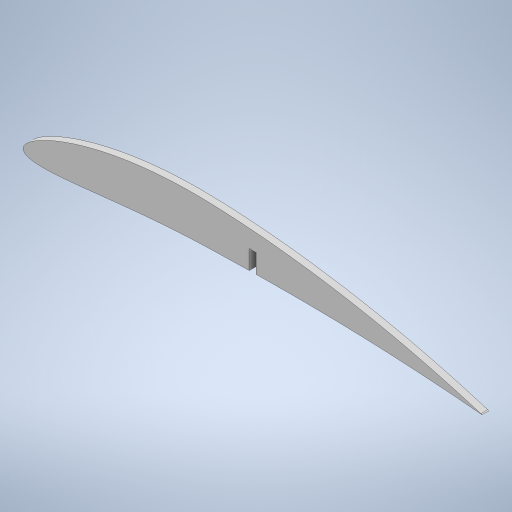
# Autodesk Inventor part: 6409_v1
Saved by Autodesk Inventor 2023 (Build 270158000, 158)
## iProperties
Created: 2023-03-24
Part Number: 6409_v1
Material: 一般
Document SubType Name: Modeling
Designer: USER
Density: 1 g/cm^3
Appearance: 預設
Author: USER
Autodesk Inventor part; units mm, degrees
ref_plane "YZ Plane" through (0, 0, 0) normal (1, 0, 0) x (0, 1, 0)
ref_plane "XZ Plane" through (0, 0, 0) normal (0, 1, 0) x (-1, 0, 0)
ref_plane "XY Plane" through (0, 0, 0) normal (0, 0, 1) x (1, 0, 0)
sketch "草圖1" plane through (0, 0, 0) normal (0, 0, 1) x (1, 0, 0)
  line L0 (0, 0) -> (200, 0)
  line L1 (199.444, 0.05) -> (200, 0)
  line L2 (199.464, 0.168) -> (200, 0)
  spline S0 degree 5 poles (199.464, 0.168) (199.4095, 0.1835) (199.2336, 0.2336) (198.9218, 0.3242) (198.496, 0.4567) (197.962, 0.6342) (197.287, 0.8521) (196.4984, 1.0928) (195.6233, 1.3514) (194.7061, 1.6209) (193.7762, 1.8964) (192.8362, 2.177) (191.8768, 2.4631) (190.8844, 2.7561) (189.8526, 3.0561) (188.7833, 3.3625) (187.6822, 3.6741) (186.5571, 3.9893) (185.4138, 4.3073) (184.2543, 4.6272) (183.0784, 4.9491) (181.8846, 5.2728) (180.6711, 5.5984) (179.4371, 5.9257) (178.183, 6.2543) (176.9101, 6.5838) (175.6203, 6.9137) (174.3152, 7.2433) (172.9962, 7.5724) (171.664, 7.9007) (170.319, 8.2281) (168.9611, 8.5544) (167.5902, 8.8796) (166.2063, 9.2036) (164.8097, 9.5262) (163.4007, 9.8473) (161.9799, 10.1664) (160.548, 10.4834) (159.1056, 10.798) (157.6531, 11.11) (156.1909, 11.4191) (154.7194, 11.7252) (153.2387, 12.0283) (151.7491, 12.3283) (150.2507, 12.6249) (148.7438, 12.9182) (147.2286, 13.208) (145.7054, 13.4942) (144.1748, 13.7765) (142.6369, 14.0549) (141.0922, 14.3291) (139.541, 14.5991) (137.9837, 14.8646) (136.4204, 15.1257) (134.8513, 15.3821) (133.2768, 15.6338) (131.6969, 15.8807) (130.1119, 16.1228) (128.5219, 16.3598) (126.9272, 16.5917) (125.328, 16.8185) (123.7244, 17.04) (122.1167, 17.256) (120.5053, 17.4666) (118.8902, 17.6716) (117.272, 17.871) (115.6509, 18.0647) (114.0273, 18.2527) (112.4014, 18.4349) (110.7734, 18.6112) (109.1437, 18.7814) (107.5123, 18.9454) (105.8794, 19.103) (104.245, 19.2542) (102.6092, 19.3986) (100.9723, 19.5363) (99.3345, 19.6671) (97.6961, 19.7913) (96.0577, 19.9087) (94.4196, 20.0198) (92.7824, 20.1244) (91.1465, 20.2228) (89.5119, 20.3148) (87.8788, 20.4002) (86.2468, 20.4787) (84.6155, 20.5496) (82.9845, 20.6124) (81.3534, 20.6662) (79.7218, 20.7103) (78.0897, 20.744) (76.4575, 20.7666) (74.8259, 20.7775) (73.1957, 20.7763) (71.5681, 20.7625) (69.9439, 20.7358) (68.3242, 20.696) (66.7097, 20.643) (65.1008, 20.5768) (63.4979, 20.4976) (61.9011, 20.4053) (60.3105, 20.3004) (58.7262, 20.1828) (57.1483, 20.0528) (55.5771, 19.9104) (54.0129, 19.7558) (52.4562, 19.5889) (50.9074, 19.4098) (49.3671, 19.2184) (47.8357, 19.0148) (46.3136, 18.7991) (44.8014, 18.5712) (43.2993, 18.3313) (41.8078, 18.0795) (40.3272, 17.816) (38.858, 17.5408) (37.4006, 17.2541) (35.9555, 16.9562) (34.5231, 16.6473) (33.1039, 16.3274) (31.6986, 15.9968) (30.3076, 15.6556) (28.9316, 15.304) (27.5711, 14.9419) (26.2267, 14.5696) (24.899, 14.1872) (23.5886, 13.7948) (22.2961, 13.3927) (21.0222, 12.9812) (19.7674, 12.5607) (18.5326, 12.1315) (17.3186, 11.6937) (16.1265, 11.2477) (14.9573, 10.7932) (13.8123, 10.3304) (12.6929, 9.8591) (11.6003, 9.3796) (10.5358, 8.8922) (9.5005, 8.3976) (8.4956, 7.8963) (7.5226, 7.3887) (6.5837, 6.8747) (5.6816, 6.3534) (4.8196, 5.8236) (4.0017, 5.2845) (3.2322, 4.7361) (2.5159, 4.1804) (1.8583, 3.6194) (1.2677, 3.0533) (0.7555, 2.4773) (0.3382, 1.8826) (0.0385, 1.2662) (-0.1096, 0.6422) (-0.0677, 0.0433) (0.1824, -0.4963) (0.6145, -0.9555) (1.1788, -1.3267) (1.8344, -1.6157) (2.5605, -1.8373) (3.3461, -2.0093) (4.1841, -2.1444) (5.0679, -2.2486) (5.9921, -2.3244) (6.9524, -2.3733) (7.9452, -2.3979) (8.968, -2.4011) (10.0186, -2.3861) (11.0953, -2.3557) (12.1964, -2.3118) (13.3204, -2.2555) (14.4661, -2.1876) (15.6322, -2.1089) (16.8177, -2.0202) (18.0217, -1.9223) (19.2436, -1.8164) (20.4826, -1.7033) (21.738, -1.584) (23.0091, -1.4593) (24.2952, -1.3298) (25.5956, -1.1961) (26.9095, -1.0586) (28.2365, -0.9178) (29.5761, -0.7742) (30.9277, -0.6281) (32.2912, -0.48) (33.6662, -0.3303) (35.0524, -0.1793) (36.4495, -0.0276) (37.857, 0.1246) (39.2746, 0.2768) (40.7019, 0.4287) (42.1384, 0.5799) (43.5837, 0.73) (45.0375, 0.8788) (46.4996, 1.0258) (47.9697, 1.1707) (49.4477, 1.3133) (50.9332, 1.4531) (52.4262, 1.59) (53.9265, 1.7237) (55.4338, 1.854) (56.948, 1.9808) (58.4688, 2.1039) (59.9958, 2.223) (61.5288, 2.338) (63.0673, 2.4485) (64.6108, 2.5544) (66.1589, 2.6552) (67.7112, 2.7507) (69.2676, 2.8408) (70.8281, 2.9251) (72.3929, 3.0037) (73.9625, 3.0764) (75.5374, 3.1435) (77.1181, 3.2051) (78.7049, 3.2615) (80.2978, 3.3131) (81.8967, 3.3604) (83.5008, 3.4042) (85.1094, 3.445) (86.7214, 3.4836) (88.3359, 3.5204) (89.952, 3.556) (91.5692, 3.5905) (93.187, 3.6238) (94.8053, 3.6559) (96.424, 3.6864) (98.0432, 3.7151) (99.6629, 3.7415) (101.2831, 3.7654) (102.9037, 3.7868) (104.5245, 3.8056) (106.1452, 3.8217) (107.7654, 3.8353) (109.385, 3.8465) (111.0035, 3.8553) (112.6206, 3.8618) (114.2361, 3.8659) (115.8498, 3.8676) (117.4615, 3.8668) (119.0711, 3.8633) (120.6783, 3.8571) (122.2829, 3.8482) (123.8848, 3.8366) (125.4837, 3.8221) (127.0794, 3.805) (128.6716, 3.7851) (130.26, 3.7626) (131.8445, 3.7374) (133.4248, 3.7096) (135.0006, 3.6791) (136.5718, 3.646) (138.1379, 3.6102) (139.6989, 3.5718) (141.2543, 3.5307) (142.8039, 3.487) (144.3475, 3.4408) (145.8845, 3.3921) (147.4148, 3.3409) (148.9381, 3.2874) (150.454, 3.2316) (151.9623, 3.1735) (153.4627, 3.1132) (154.9551, 3.0506) (156.4392, 2.9857) (157.9145, 2.9187) (159.3809, 2.8495) (160.8377, 2.7784) (162.2844, 2.7053) (163.7204, 2.6305) (165.1452, 2.5541) (166.5583, 2.4763) (167.9594, 2.3969) (169.3483, 2.3162) (170.7249, 2.2339) (172.0891, 2.1502) (173.4403, 2.0649) (174.778, 1.9784) (176.1009, 1.8908) (177.4074, 1.8025) (178.6961, 1.714) (179.9659, 1.6254) (181.2162, 1.5369) (182.4477, 1.4482) (183.6617, 1.359) (184.8595, 1.2688) (186.0408, 1.1775) (187.2035, 1.0856) (188.3417, 0.9942) (189.4483, 0.9051) (190.5176, 0.8193) (191.5476, 0.7372) (192.5445, 0.6572) (193.521, 0.5757) (194.4856, 0.4907) (195.4358, 0.4023) (196.3428, 0.3174) (197.1637, 0.246) (197.8722, 0.1935) (198.4359, 0.1544) (198.8815, 0.1138) (199.2051, 0.0778) (199.3872, 0.0567) (199.444, 0.05) knots 0.005109 0.005109 0.005109 0.005109 0.005109 0.005109 0.006667 0.01 0.013333 0.016667 0.02 0.023333 0.026667 0.03 0.033333 0.036667 0.04 0.043333 0.046667 0.05 0.053333 0.056667 0.06 0.063333 0.066667 0.07 0.073333 0.076667 0.08 0.083333 0.086667 0.09 0.093333 0.096667 0.1 0.103333 0.106667 0.11 0.113333 0.116667 0.12 0.123333 0.126667 0.13 0.133333 0.136667 0.14 0.143333 0.146667 0.15 0.153333 0.156667 0.16 0.163333 0.166667 0.17 0.173333 0.176667 0.18 0.183333 0.186667 0.19 0.193333 0.196667 0.2 0.203333 0.206667 0.21 0.213333 0.216667 0.22 0.223333 0.226667 0.23 0.233333 0.236667 0.24 0.243333 0.246667 0.25 0.253333 0.256667 0.26 0.263333 0.266667 0.27 0.273333 0.276667 0.28 0.283333 0.286667 0.29 0.293333 0.296667 0.3 0.303333 0.306667 0.31 0.313333 0.316667 0.32 0.323333 0.326667 0.33 0.333333 0.336667 0.34 0.343333 0.346667 0.35 0.353333 0.356667 0.36 0.363333 0.366667 0.37 0.373333 0.376667 0.38 0.383333 0.386667 0.39 0.393333 0.396667 0.4 0.403333 0.406667 0.41 0.413333 0.416667 0.42 0.423333 0.426667 0.43 0.433333 0.436667 0.44 0.443333 0.446667 0.45 0.453333 0.456667 0.46 0.463333 0.466667 0.47 0.473333 0.476667 0.48 0.483333 0.486667 0.49 0.493333 0.496667 0.5 0.503333 0.506667 0.51 0.513333 0.516667 0.52 0.523333 0.526667 0.53 0.533333 0.536667 0.54 0.543333 0.546667 0.55 0.553333 0.556667 0.56 0.563333 0.566667 0.57 0.573333 0.576667 0.58 0.583333 0.586667 0.59 0.593333 0.596667 0.6 0.603333 0.606667 0.61 0.613333 0.616667 0.62 0.623333 0.626667 0.63 0.633333 0.636667 0.64 0.643333 0.646667 0.65 0.653333 0.656667 0.66 0.663333 0.666667 0.67 0.673333 0.676667 0.68 0.683333 0.686667 0.69 0.693333 0.696667 0.7 0.703333 0.706667 0.71 0.713333 0.716667 0.72 0.723333 0.726667 0.73 0.733333 0.736667 0.74 0.743333 0.746667 0.75 0.753333 0.756667 0.76 0.763333 0.766667 0.77 0.773333 0.776667 0.78 0.783333 0.786667 0.79 0.793333 0.796667 0.8 0.803333 0.806667 0.81 0.813333 0.816667 0.82 0.823333 0.826667 0.83 0.833333 0.836667 0.84 0.843333 0.846667 0.85 0.853333 0.856667 0.86 0.863333 0.866667 0.87 0.873333 0.876667 0.88 0.883333 0.886667 0.89 0.893333 0.896667 0.9 0.903333 0.906667 0.91 0.913333 0.916667 0.92 0.923333 0.926667 0.93 0.933333 0.936667 0.94 0.943333 0.946667 0.95 0.953333 0.956667 0.96 0.963333 0.966667 0.97 0.973333 0.976667 0.98 0.983333 0.986667 0.99 0.993333 0.994906 0.994906 0.994906 0.994906 0.994906 0.994906 weights 1 1 1 1 1 1 1 1 1 1 1 1 1 1 1 1 1 1 1 1 1 1 1 1 1 1 1 1 1 1 1 1 1 1 1 1 1 1 1 1 1 1 1 1 1 1 1 1 1 1 1 1 1 1 1 1 1 1 1 1 1 1 1 1 1 1 1 1 1 1 1 1 1 1 1 1 1 1 1 1 1 1 1 1 1 1 1 1 1 1 1 1 1 1 1 1 1 1 1 1 1 1 1 1 1 1 1 1 1 1 1 1 1 1 1 1 1 1 1 1 1 1 1 1 1 1 1 1 1 1 1 1 1 1 1 1 1 1 1 1 1 1 1 1 1 1 1 1 1 1 1 1 1 1 1 1 1 1 1 1 1 1 1 1 1 1 1 1 1 1 1 1 1 1 1 1 1 1 1 1 1 1 1 1 1 1 1 1 1 1 1 1 1 1 1 1 1 1 1 1 1 1 1 1 1 1 1 1 1 1 1 1 1 1 1 1 1 1 1 1 1 1 1 1 1 1 1 1 1 1 1 1 1 1 1 1 1 1 1 1 1 1 1 1 1 1 1 1 1 1 1 1 1 1 1 1 1 1 1 1 1 1 1 1 1 1 1 1 1 1 1 1 1 1 1 1 1 1 1 1 1 1 1 1 1 1 1 1 1 1 1 1 1 1 1 1 1 1 1 1 1 1 1
  line L3 (199.464, 0.168) -> (199.4095, 0.1835) construction
  line L4 (199.4095, 0.1835) -> (199.2336, 0.2336) construction
  line L5 (199.2336, 0.2336) -> (198.9218, 0.3242) construction
  line L6 (198.9218, 0.3242) -> (198.496, 0.4567) construction
  line L7 (198.496, 0.4567) -> (197.962, 0.6342) construction
  line L8 (197.962, 0.6342) -> (197.287, 0.8521) construction
  line L9 (197.287, 0.8521) -> (196.4984, 1.0928) construction
  line L10 (196.4984, 1.0928) -> (195.6233, 1.3514) construction
  line L11 (195.6233, 1.3514) -> (194.7061, 1.6209) construction
  line L12 (194.7061, 1.6209) -> (193.7762, 1.8964) construction
  line L13 (193.7762, 1.8964) -> (192.8362, 2.177) construction
  line L14 (192.8362, 2.177) -> (191.8768, 2.4631) construction
  line L15 (191.8768, 2.4631) -> (190.8844, 2.7561) construction
  line L16 (190.8844, 2.7561) -> (189.8526, 3.0561) construction
  line L17 (189.8526, 3.0561) -> (188.7833, 3.3625) construction
  line L18 (188.7833, 3.3625) -> (187.6822, 3.6741) construction
  line L19 (187.6822, 3.6741) -> (186.5571, 3.9893) construction
  line L20 (186.5571, 3.9893) -> (185.4138, 4.3073) construction
  line L21 (185.4138, 4.3073) -> (184.2543, 4.6272) construction
  line L22 (184.2543, 4.6272) -> (183.0784, 4.9491) construction
  line L23 (183.0784, 4.9491) -> (181.8846, 5.2728) construction
  line L24 (181.8846, 5.2728) -> (180.6711, 5.5984) construction
  line L25 (180.6711, 5.5984) -> (179.4371, 5.9257) construction
  line L26 (179.4371, 5.9257) -> (178.183, 6.2543) construction
  line L27 (178.183, 6.2543) -> (176.9101, 6.5838) construction
  line L28 (176.9101, 6.5838) -> (175.6203, 6.9137) construction
  line L29 (175.6203, 6.9137) -> (174.3152, 7.2433) construction
  line L30 (174.3152, 7.2433) -> (172.9962, 7.5724) construction
  line L31 (172.9962, 7.5724) -> (171.664, 7.9007) construction
  line L32 (171.664, 7.9007) -> (170.319, 8.2281) construction
  line L33 (170.319, 8.2281) -> (168.9611, 8.5544) construction
  line L34 (168.9611, 8.5544) -> (167.5902, 8.8796) construction
  line L35 (167.5902, 8.8796) -> (166.2063, 9.2036) construction
  line L36 (166.2063, 9.2036) -> (164.8097, 9.5262) construction
  line L37 (164.8097, 9.5262) -> (163.4007, 9.8473) construction
  line L38 (163.4007, 9.8473) -> (161.9799, 10.1664) construction
  line L39 (161.9799, 10.1664) -> (160.548, 10.4834) construction
  line L40 (160.548, 10.4834) -> (159.1056, 10.798) construction
  line L41 (159.1056, 10.798) -> (157.6531, 11.11) construction
  line L42 (157.6531, 11.11) -> (156.1909, 11.4191) construction
  line L43 (156.1909, 11.4191) -> (154.7194, 11.7252) construction
  line L44 (154.7194, 11.7252) -> (153.2387, 12.0283) construction
  line L45 (153.2387, 12.0283) -> (151.7491, 12.3283) construction
  line L46 (151.7491, 12.3283) -> (150.2507, 12.6249) construction
  line L47 (150.2507, 12.6249) -> (148.7438, 12.9182) construction
  line L48 (148.7438, 12.9182) -> (147.2286, 13.208) construction
  line L49 (147.2286, 13.208) -> (145.7054, 13.4942) construction
  line L50 (145.7054, 13.4942) -> (144.1748, 13.7765) construction
  line L51 (144.1748, 13.7765) -> (142.6369, 14.0549) construction
  line L52 (142.6369, 14.0549) -> (141.0922, 14.3291) construction
  line L53 (141.0922, 14.3291) -> (139.541, 14.5991) construction
  line L54 (139.541, 14.5991) -> (137.9837, 14.8646) construction
  line L55 (137.9837, 14.8646) -> (136.4204, 15.1257) construction
  line L56 (136.4204, 15.1257) -> (134.8513, 15.3821) construction
  line L57 (134.8513, 15.3821) -> (133.2768, 15.6338) construction
  line L58 (133.2768, 15.6338) -> (131.6969, 15.8807) construction
  line L59 (131.6969, 15.8807) -> (130.1119, 16.1228) construction
  line L60 (130.1119, 16.1228) -> (128.5219, 16.3598) construction
  line L61 (128.5219, 16.3598) -> (126.9272, 16.5917) construction
  line L62 (126.9272, 16.5917) -> (125.328, 16.8185) construction
  line L63 (125.328, 16.8185) -> (123.7244, 17.04) construction
  line L64 (123.7244, 17.04) -> (122.1167, 17.256) construction
  line L65 (122.1167, 17.256) -> (120.5053, 17.4666) construction
  line L66 (120.5053, 17.4666) -> (118.8902, 17.6716) construction
  line L67 (118.8902, 17.6716) -> (117.272, 17.871) construction
  line L68 (117.272, 17.871) -> (115.6509, 18.0647) construction
  line L69 (115.6509, 18.0647) -> (114.0273, 18.2527) construction
  line L70 (114.0273, 18.2527) -> (112.4014, 18.4349) construction
  line L71 (112.4014, 18.4349) -> (110.7734, 18.6112) construction
  line L72 (110.7734, 18.6112) -> (109.1437, 18.7814) construction
  line L73 (109.1437, 18.7814) -> (107.5123, 18.9454) construction
  line L74 (107.5123, 18.9454) -> (105.8794, 19.103) construction
  line L75 (105.8794, 19.103) -> (104.245, 19.2542) construction
  line L76 (104.245, 19.2542) -> (102.6092, 19.3986) construction
  line L77 (102.6092, 19.3986) -> (100.9723, 19.5363) construction
  line L78 (100.9723, 19.5363) -> (99.3345, 19.6671) construction
  line L79 (99.3345, 19.6671) -> (97.6961, 19.7913) construction
  line L80 (97.6961, 19.7913) -> (96.0577, 19.9087) construction
  line L81 (96.0577, 19.9087) -> (94.4196, 20.0198) construction
  line L82 (94.4196, 20.0198) -> (92.7824, 20.1244) construction
  line L83 (92.7824, 20.1244) -> (91.1465, 20.2228) construction
  line L84 (91.1465, 20.2228) -> (89.5119, 20.3148) construction
  line L85 (89.5119, 20.3148) -> (87.8788, 20.4002) construction
  line L86 (87.8788, 20.4002) -> (86.2468, 20.4787) construction
  line L87 (86.2468, 20.4787) -> (84.6155, 20.5496) construction
  line L88 (84.6155, 20.5496) -> (82.9845, 20.6124) construction
  line L89 (82.9845, 20.6124) -> (81.3534, 20.6662) construction
  line L90 (81.3534, 20.6662) -> (79.7218, 20.7103) construction
  line L91 (79.7218, 20.7103) -> (78.0897, 20.744) construction
  line L92 (78.0897, 20.744) -> (76.4575, 20.7666) construction
  line L93 (76.4575, 20.7666) -> (74.8259, 20.7775) construction
  line L94 (74.8259, 20.7775) -> (73.1957, 20.7763) construction
  line L95 (73.1957, 20.7763) -> (71.5681, 20.7625) construction
  line L96 (71.5681, 20.7625) -> (69.9439, 20.7358) construction
  line L97 (69.9439, 20.7358) -> (68.3242, 20.696) construction
  line L98 (68.3242, 20.696) -> (66.7097, 20.643) construction
  line L99 (66.7097, 20.643) -> (65.1008, 20.5768) construction
  line L100 (65.1008, 20.5768) -> (63.4979, 20.4976) construction
  line L101 (63.4979, 20.4976) -> (61.9011, 20.4053) construction
  line L102 (61.9011, 20.4053) -> (60.3105, 20.3004) construction
  line L103 (60.3105, 20.3004) -> (58.7262, 20.1828) construction
  line L104 (58.7262, 20.1828) -> (57.1483, 20.0528) construction
  line L105 (57.1483, 20.0528) -> (55.5771, 19.9104) construction
  line L106 (55.5771, 19.9104) -> (54.0129, 19.7558) construction
  line L107 (54.0129, 19.7558) -> (52.4562, 19.5889) construction
  line L108 (52.4562, 19.5889) -> (50.9074, 19.4098) construction
  line L109 (50.9074, 19.4098) -> (49.3671, 19.2184) construction
  line L110 (49.3671, 19.2184) -> (47.8357, 19.0148) construction
  line L111 (47.8357, 19.0148) -> (46.3136, 18.7991) construction
  line L112 (46.3136, 18.7991) -> (44.8014, 18.5712) construction
  line L113 (44.8014, 18.5712) -> (43.2993, 18.3313) construction
  line L114 (43.2993, 18.3313) -> (41.8078, 18.0795) construction
  line L115 (41.8078, 18.0795) -> (40.3272, 17.816) construction
  line L116 (40.3272, 17.816) -> (38.858, 17.5408) construction
  line L117 (38.858, 17.5408) -> (37.4006, 17.2541) construction
  line L118 (37.4006, 17.2541) -> (35.9555, 16.9562) construction
  line L119 (35.9555, 16.9562) -> (34.5231, 16.6473) construction
  line L120 (34.5231, 16.6473) -> (33.1039, 16.3274) construction
  line L121 (33.1039, 16.3274) -> (31.6986, 15.9968) construction
  line L122 (31.6986, 15.9968) -> (30.3076, 15.6556) construction
  line L123 (30.3076, 15.6556) -> (28.9316, 15.304) construction
  line L124 (28.9316, 15.304) -> (27.5711, 14.9419) construction
  line L125 (27.5711, 14.9419) -> (26.2267, 14.5696) construction
  line L126 (26.2267, 14.5696) -> (24.899, 14.1872) construction
  line L127 (24.899, 14.1872) -> (23.5886, 13.7948) construction
  line L128 (23.5886, 13.7948) -> (22.2961, 13.3927) construction
  line L129 (22.2961, 13.3927) -> (21.0222, 12.9812) construction
  line L130 (21.0222, 12.9812) -> (19.7674, 12.5607) construction
  line L131 (19.7674, 12.5607) -> (18.5326, 12.1315) construction
  line L132 (18.5326, 12.1315) -> (17.3186, 11.6937) construction
  line L133 (17.3186, 11.6937) -> (16.1265, 11.2477) construction
  line L134 (16.1265, 11.2477) -> (14.9573, 10.7932) construction
  line L135 (14.9573, 10.7932) -> (13.8123, 10.3304) construction
  line L136 (13.8123, 10.3304) -> (12.6929, 9.8591) construction
  line L137 (12.6929, 9.8591) -> (11.6003, 9.3796) construction
  line L138 (11.6003, 9.3796) -> (10.5358, 8.8922) construction
  line L139 (10.5358, 8.8922) -> (9.5005, 8.3976) construction
  line L140 (9.5005, 8.3976) -> (8.4956, 7.8963) construction
  line L141 (8.4956, 7.8963) -> (7.5226, 7.3887) construction
  line L142 (7.5226, 7.3887) -> (6.5837, 6.8747) construction
  line L143 (6.5837, 6.8747) -> (5.6816, 6.3534) construction
  line L144 (5.6816, 6.3534) -> (4.8196, 5.8236) construction
  line L145 (4.8196, 5.8236) -> (4.0017, 5.2845) construction
  line L146 (4.0017, 5.2845) -> (3.2322, 4.7361) construction
  line L147 (3.2322, 4.7361) -> (2.5159, 4.1804) construction
  line L148 (2.5159, 4.1804) -> (1.8583, 3.6194) construction
  line L149 (1.8583, 3.6194) -> (1.2677, 3.0533) construction
  line L150 (1.2677, 3.0533) -> (0.7555, 2.4773) construction
  line L151 (0.7555, 2.4773) -> (0.3382, 1.8826) construction
  line L152 (0.3382, 1.8826) -> (0.0385, 1.2662) construction
  line L153 (0.0385, 1.2662) -> (-0.1096, 0.6422) construction
  line L154 (-0.1096, 0.6422) -> (-0.0677, 0.0433) construction
  line L155 (-0.0677, 0.0433) -> (0.1824, -0.4963) construction
  line L156 (0.1824, -0.4963) -> (0.6145, -0.9555) construction
  line L157 (0.6145, -0.9555) -> (1.1788, -1.3267) construction
  line L158 (1.1788, -1.3267) -> (1.8344, -1.6157) construction
  line L159 (1.8344, -1.6157) -> (2.5605, -1.8373) construction
  line L160 (2.5605, -1.8373) -> (3.3461, -2.0093) construction
  line L161 (3.3461, -2.0093) -> (4.1841, -2.1444) construction
  line L162 (4.1841, -2.1444) -> (5.0679, -2.2486) construction
  line L163 (5.0679, -2.2486) -> (5.9921, -2.3244) construction
  line L164 (5.9921, -2.3244) -> (6.9524, -2.3733) construction
  line L165 (6.9524, -2.3733) -> (7.9452, -2.3979) construction
  line L166 (7.9452, -2.3979) -> (8.968, -2.4011) construction
  line L167 (8.968, -2.4011) -> (10.0186, -2.3861) construction
  line L168 (10.0186, -2.3861) -> (11.0953, -2.3557) construction
  line L169 (11.0953, -2.3557) -> (12.1964, -2.3118) construction
  line L170 (12.1964, -2.3118) -> (13.3204, -2.2555) construction
  line L171 (13.3204, -2.2555) -> (14.4661, -2.1876) construction
  line L172 (14.4661, -2.1876) -> (15.6322, -2.1089) construction
  line L173 (15.6322, -2.1089) -> (16.8177, -2.0202) construction
  line L174 (16.8177, -2.0202) -> (18.0217, -1.9223) construction
  line L175 (18.0217, -1.9223) -> (19.2436, -1.8164) construction
  line L176 (19.2436, -1.8164) -> (20.4826, -1.7033) construction
  line L177 (20.4826, -1.7033) -> (21.738, -1.584) construction
  line L178 (21.738, -1.584) -> (23.0091, -1.4593) construction
  line L179 (23.0091, -1.4593) -> (24.2952, -1.3298) construction
  line L180 (24.2952, -1.3298) -> (25.5956, -1.1961) construction
  line L181 (25.5956, -1.1961) -> (26.9095, -1.0586) construction
  line L182 (26.9095, -1.0586) -> (28.2365, -0.9178) construction
  line L183 (28.2365, -0.9178) -> (29.5761, -0.7742) construction
  line L184 (29.5761, -0.7742) -> (30.9277, -0.6281) construction
  line L185 (30.9277, -0.6281) -> (32.2912, -0.48) construction
  line L186 (32.2912, -0.48) -> (33.6662, -0.3303) construction
  line L187 (33.6662, -0.3303) -> (35.0524, -0.1793) construction
  line L188 (35.0524, -0.1793) -> (36.4495, -0.0276) construction
  line L189 (36.4495, -0.0276) -> (37.857, 0.1246) construction
  line L190 (37.857, 0.1246) -> (39.2746, 0.2768) construction
  line L191 (39.2746, 0.2768) -> (40.7019, 0.4287) construction
  line L192 (40.7019, 0.4287) -> (42.1384, 0.5799) construction
  line L193 (42.1384, 0.5799) -> (43.5837, 0.73) construction
  line L194 (43.5837, 0.73) -> (45.0375, 0.8788) construction
  line L195 (45.0375, 0.8788) -> (46.4996, 1.0258) construction
  line L196 (46.4996, 1.0258) -> (47.9697, 1.1707) construction
  line L197 (47.9697, 1.1707) -> (49.4477, 1.3133) construction
  line L198 (49.4477, 1.3133) -> (50.9332, 1.4531) construction
  line L199 (50.9332, 1.4531) -> (52.4262, 1.59) construction
  line L200 (52.4262, 1.59) -> (53.9265, 1.7237) construction
  line L201 (53.9265, 1.7237) -> (55.4338, 1.854) construction
  line L202 (55.4338, 1.854) -> (56.948, 1.9808) construction
  line L203 (56.948, 1.9808) -> (58.4688, 2.1039) construction
  line L204 (58.4688, 2.1039) -> (59.9958, 2.223) construction
  line L205 (59.9958, 2.223) -> (61.5288, 2.338) construction
  line L206 (61.5288, 2.338) -> (63.0673, 2.4485) construction
  line L207 (63.0673, 2.4485) -> (64.6108, 2.5544) construction
  line L208 (64.6108, 2.5544) -> (66.1589, 2.6552) construction
  line L209 (66.1589, 2.6552) -> (67.7112, 2.7507) construction
  line L210 (67.7112, 2.7507) -> (69.2676, 2.8408) construction
  line L211 (69.2676, 2.8408) -> (70.8281, 2.9251) construction
  line L212 (70.8281, 2.9251) -> (72.3929, 3.0037) construction
  line L213 (72.3929, 3.0037) -> (73.9625, 3.0764) construction
  line L214 (73.9625, 3.0764) -> (75.5374, 3.1435) construction
  line L215 (75.5374, 3.1435) -> (77.1181, 3.2051) construction
  line L216 (77.1181, 3.2051) -> (78.7049, 3.2615) construction
  line L217 (78.7049, 3.2615) -> (80.2978, 3.3131) construction
  line L218 (80.2978, 3.3131) -> (81.8967, 3.3604) construction
  line L219 (81.8967, 3.3604) -> (83.5008, 3.4042) construction
  line L220 (83.5008, 3.4042) -> (85.1094, 3.445) construction
  line L221 (85.1094, 3.445) -> (86.7214, 3.4836) construction
  line L222 (86.7214, 3.4836) -> (88.3359, 3.5204) construction
  line L223 (88.3359, 3.5204) -> (89.952, 3.556) construction
  line L224 (89.952, 3.556) -> (91.5692, 3.5905) construction
  line L225 (91.5692, 3.5905) -> (93.187, 3.6238) construction
  line L226 (93.187, 3.6238) -> (94.8053, 3.6559) construction
  line L227 (94.8053, 3.6559) -> (96.424, 3.6864) construction
  line L228 (96.424, 3.6864) -> (98.0432, 3.7151) construction
  line L229 (98.0432, 3.7151) -> (99.6629, 3.7415) construction
  line L230 (99.6629, 3.7415) -> (101.2831, 3.7654) construction
  line L231 (101.2831, 3.7654) -> (102.9037, 3.7868) construction
  line L232 (102.9037, 3.7868) -> (104.5245, 3.8056) construction
  line L233 (104.5245, 3.8056) -> (106.1452, 3.8217) construction
  line L234 (106.1452, 3.8217) -> (107.7654, 3.8353) construction
  line L235 (107.7654, 3.8353) -> (109.385, 3.8465) construction
  line L236 (109.385, 3.8465) -> (111.0035, 3.8553) construction
  line L237 (111.0035, 3.8553) -> (112.6206, 3.8618) construction
  line L238 (112.6206, 3.8618) -> (114.2361, 3.8659) construction
  line L239 (114.2361, 3.8659) -> (115.8498, 3.8676) construction
  line L240 (115.8498, 3.8676) -> (117.4615, 3.8668) construction
  line L241 (117.4615, 3.8668) -> (119.0711, 3.8633) construction
  line L242 (119.0711, 3.8633) -> (120.6783, 3.8571) construction
  line L243 (120.6783, 3.8571) -> (122.2829, 3.8482) construction
  line L244 (122.2829, 3.8482) -> (123.8848, 3.8366) construction
  line L245 (123.8848, 3.8366) -> (125.4837, 3.8221) construction
  line L246 (125.4837, 3.8221) -> (127.0794, 3.805) construction
  line L247 (127.0794, 3.805) -> (128.6716, 3.7851) construction
  line L248 (128.6716, 3.7851) -> (130.26, 3.7626) construction
  line L249 (130.26, 3.7626) -> (131.8445, 3.7374) construction
  line L250 (131.8445, 3.7374) -> (133.4248, 3.7096) construction
  line L251 (133.4248, 3.7096) -> (135.0006, 3.6791) construction
  line L252 (135.0006, 3.6791) -> (136.5718, 3.646) construction
  line L253 (136.5718, 3.646) -> (138.1379, 3.6102) construction
  line L254 (138.1379, 3.6102) -> (139.6989, 3.5718) construction
  line L255 (139.6989, 3.5718) -> (141.2543, 3.5307) construction
  line L256 (141.2543, 3.5307) -> (142.8039, 3.487) construction
  line L257 (142.8039, 3.487) -> (144.3475, 3.4408) construction
  line L258 (144.3475, 3.4408) -> (145.8845, 3.3921) construction
  line L259 (145.8845, 3.3921) -> (147.4148, 3.3409) construction
  line L260 (147.4148, 3.3409) -> (148.9381, 3.2874) construction
  line L261 (148.9381, 3.2874) -> (150.454, 3.2316) construction
  line L262 (150.454, 3.2316) -> (151.9623, 3.1735) construction
  line L263 (151.9623, 3.1735) -> (153.4627, 3.1132) construction
  line L264 (153.4627, 3.1132) -> (154.9551, 3.0506) construction
  line L265 (154.9551, 3.0506) -> (156.4392, 2.9857) construction
  line L266 (156.4392, 2.9857) -> (157.9145, 2.9187) construction
  line L267 (157.9145, 2.9187) -> (159.3809, 2.8495) construction
  line L268 (159.3809, 2.8495) -> (160.8377, 2.7784) construction
  line L269 (160.8377, 2.7784) -> (162.2844, 2.7053) construction
  line L270 (162.2844, 2.7053) -> (163.7204, 2.6305) construction
  line L271 (163.7204, 2.6305) -> (165.1452, 2.5541) construction
  line L272 (165.1452, 2.5541) -> (166.5583, 2.4763) construction
  line L273 (166.5583, 2.4763) -> (167.9594, 2.3969) construction
  line L274 (167.9594, 2.3969) -> (169.3483, 2.3162) construction
  line L275 (169.3483, 2.3162) -> (170.7249, 2.2339) construction
  line L276 (170.7249, 2.2339) -> (172.0891, 2.1502) construction
  line L277 (172.0891, 2.1502) -> (173.4403, 2.0649) construction
  line L278 (173.4403, 2.0649) -> (174.778, 1.9784) construction
  line L279 (174.778, 1.9784) -> (176.1009, 1.8908) construction
  line L280 (176.1009, 1.8908) -> (177.4074, 1.8025) construction
  line L281 (177.4074, 1.8025) -> (178.6961, 1.714) construction
  line L282 (178.6961, 1.714) -> (179.9659, 1.6254) construction
  line L283 (179.9659, 1.6254) -> (181.2162, 1.5369) construction
  line L284 (181.2162, 1.5369) -> (182.4477, 1.4482) construction
  line L285 (182.4477, 1.4482) -> (183.6617, 1.359) construction
  line L286 (183.6617, 1.359) -> (184.8595, 1.2688) construction
  line L287 (184.8595, 1.2688) -> (186.0408, 1.1775) construction
  line L288 (186.0408, 1.1775) -> (187.2035, 1.0856) construction
  line L289 (187.2035, 1.0856) -> (188.3417, 0.9942) construction
  line L290 (188.3417, 0.9942) -> (189.4483, 0.9051) construction
  line L291 (189.4483, 0.9051) -> (190.5176, 0.8193) construction
  line L292 (190.5176, 0.8193) -> (191.5476, 0.7372) construction
  line L293 (191.5476, 0.7372) -> (192.5445, 0.6572) construction
  line L294 (192.5445, 0.6572) -> (193.521, 0.5757) construction
  line L295 (193.521, 0.5757) -> (194.4856, 0.4907) construction
  line L296 (194.4856, 0.4907) -> (195.4358, 0.4023) construction
  line L297 (195.4358, 0.4023) -> (196.3428, 0.3174) construction
  line L298 (196.3428, 0.3174) -> (197.1637, 0.246) construction
  line L299 (197.1637, 0.246) -> (197.8722, 0.1935) construction
  line L300 (197.8722, 0.1935) -> (198.4359, 0.1544) construction
  line L301 (198.4359, 0.1544) -> (198.8815, 0.1138) construction
  line L302 (198.8815, 0.1138) -> (199.2051, 0.0778) construction
  line L303 (199.2051, 0.0778) -> (199.3872, 0.0567) construction
  line L304 (199.3872, 0.0567) -> (199.444, 0.05) construction
  point P0 (199.444, 0.05)
  constraints: 6 end point, 2 other
extrude "擠出1" add sketch "草圖1" along normal blind 3 contours S0 L2 L1 L0 | L0 S0
sketch "草圖2" plane through (0, 0, 3) normal (0, 0, 1) x (1, 0, 0)
  line L0 (98.5, 12) -> (101.5, 12)
  line L1 (101.5, 12) -> (101.5, -5)
  line L2 (101.5, -5) -> (98.5, -5)
  line L3 (98.5, -5) -> (98.5, 12)
  line L4 (-40.1316, 0) -> (240.0219, 0) projected
  point P0 (0, 0)
  point P1 (100, 12)
  dimension "d2" = 3
  dimension "d3" = 100
  dimension "d4" = 12
  dimension "d5" = 17
  constraints: 8 end point, 2 parallel, 1 horizontal, 1 midpoint, 1 perpendicular
  measures "d2" distance of L1.end L2.end
  measures "d3" horizontal distance of point (0, 0) point (100, 12)
  measures "d4" distance from line of L4 point (100, 12)
  measures "d5" distance between parallel lines of L0 L2
extrude "擠出2" cut sketch "草圖2" against normal blind 3
